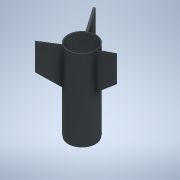
# Autodesk Inventor part: tail
Saved by Autodesk Inventor 2020.3 (Build 243373000, 373)
## iProperties
Created: 2021-01-23
Part Number: tail
Material: ABS Plastic
Document SubType Name: Modeling
Designer: 0x6f736f646f
Density: 1.06 g/cm^3
Appearance: Iron Gray
Author: 0x6f736f646f
Autodesk Inventor part; units mm, degrees
ref_plane "YZ Plane" through (0, 0, 0) normal (1, 0, 0) x (0, 1, 0)
ref_plane "XZ Plane" through (0, 0, 0) normal (0, 1, 0) x (-1, 0, 0)
ref_plane "XY Plane" through (0, 0, 0) normal (0, 0, 1) x (1, 0, 0)
sketch "Sketch1" plane through (0, 0, 0) normal (0, 1, 0) x (-1, 0, 0)
  circle A0 centre (0, 0) radius 25
  circle A1 centre (0, 0) radius 25.9
  circle A2 centre (0, 0) radius 26.8
  dimension "d0" = 50
  dimension "d1" = 51.8
  dimension "d2" = 53.6
  constraints: 3 centre point, 3 coincident
  measures "d0" diameter of A0
  measures "d1" diameter of A1
  measures "d2" diameter of A2
extrude "Extrusion1" add sketch "Sketch1" along normal blind 75 and the other way blind 80 contours A1
extrude "Extrusion2" add sketch "Sketch1" along normal blind 75 and the other way blind 75 contours A2
sketch "Sketch4" plane through (0, 0, 0) normal (0, 0, 1) x (1, 0, 0)
  line L0 (65, 99.9302) -> (65, 38.564)
  line L1 (65, 38.564) -> (25, 5)
  line L2 (25, 5) -> (25, 75)
  line L3 (25, 75) -> (65, 88.564)
  line L4 (65, 88.564) -> (65, 99.9302)
  line L5 (-25, 75) -> (25, 75) projected
  line L6 (-25, 75) -> (25, 75) projected
  line L7 (25.9, -80) -> (25, -80) projected
  line L8 (25, -80) -> (25, 75) projected
  line L9 (26.8, 75) -> (26.8, -75) projected
  line L10 (-25, -80) -> (-25.9, -80) projected
  line L11 (-26.8, -75) -> (-26.8, 75) projected
  line L12 (-25, 75) -> (-25, -80) projected
  line L13 (25, 75) -> (26.8, 75) projected
  line L14 (-26.8, 75) -> (-25, 75) projected
  line L15 (26.8, -75) -> (25.9, -75) projected
  line L16 (25.9, -75) -> (25.9, -80) projected
  line L17 (-25.9, -80) -> (-25.9, -75) projected
  line L18 (-25.9, -75) -> (-26.8, -75) projected
  point P0 (0, 0)
  point P1 (26.8, 96)
  point P2 (-26.8, 96)
  point P3 (26.8, 6.5104)
  point P4 (15.9, -100)
  point P5 (-15.9, -100)
  point P6 (25, 5)
  dimension "d18" = 70
  dimension "d21" = 50
  dimension "d24" = 50
  dimension "d25" = 40
  constraints: 10 end point, 2 vertical, 1 coincident, 1 parallel, 1 point on line
  measures "d18" distance of L2.end L1.end
  measures "d21" angle of L2 L1
  measures "d24" distance of L3.end L0.end
  measures "d25" distance between parallel lines of L8 L0
extrude "Extrusion4" add sketch "Sketch4" along normal mid plane 3.6 contours L0 L1 L9 L13 L3 | L13 L9 L1 L2 | L9 L15 L16 L7 L8 L1
pattern_circular "Circular Pattern2" count 3 over 360 about axis through (0, -10, 0) along (0, 1, 0) of "Extrusion4"
body "Solid1"
